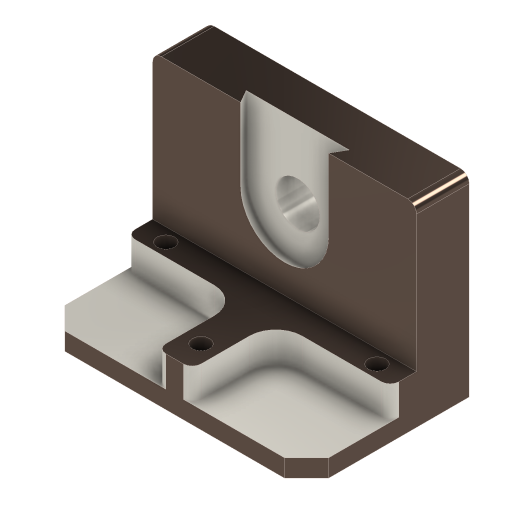
# Autodesk Inventor part: Part019. Corner block
Saved by Autodesk Inventor 2023.2 (Build 272271030, 271C)
## iProperties
Created: 2023-09-20
Part Number: Part019. Corner block
Material: Steel, Carbon
Document SubType Name: Modeling
Designer: User
Mass: 2416.08 g
Surface Area: 476.682 cm^2
Volume: 307.781 cm^3
Density: 7.85 g/cm^3
Appearance: Gunmetal - Antique Polished
Author: User
Autodesk Inventor part; units mm, degrees
ref_plane "YZ Plane" through (0, 0, 0) normal (1, 0, 0) x (0, 1, 0)
ref_plane "XZ Plane" through (0, 0, 0) normal (0, 1, 0) x (-1, 0, 0)
ref_plane "XY Plane" through (0, 0, 0) normal (0, 0, 1) x (1, 0, 0)
sketch "Sketch1" plane through (0, 0, 0) normal (0, 1, 0) x (-1, 0, 0)
  line L0 (60, -74) -> (-60, -74)
  line L1 (-60, -74) -> (-60, 0)
  line L2 (-60, 0) -> (60, 0)
  line L3 (60, 0) -> (60, -74)
  point P0 (0, 0)
  point P1 (0, 0)
  dimension "d0" = 120
  dimension "d1" = 74
  constraints: 8 end point, 2 parallel, 1 coincident, 1 horizontal, 1 midpoint, 1 perpendicular
  measures "d0" distance of L1.end L2.end
  measures "d1" distance of L0.end L1.end
extrude "Extrusion1" add sketch "Sketch1" along normal blind 8
chamfer "Chamfer1" distance 10 angle 45 2 edges at (60, 4, 0) (-60, 4, 0)
sketch "Sketch2" plane through (0, 8, 0) normal (0, 1, 0) x (1, 0, 0)
  line L0 (-50, 0) -> (-60, 10) projected
  line L1 (-50, 0) -> (50, 0) projected
  line L2 (60, 10) -> (60, 74) projected
  line L3 (60, 74) -> (-60, 74) projected
  line L4 (-60, 74) -> (-60, 10) projected
  line L5 (-60, 38) -> (-20, 38)
  line L6 (-8, 26) -> (-8, 0)
  line L7 (-8, 0) -> (-50, 0)
  line L8 (-60, 10) -> (-60, 38)
  arc A0 (-8, 26) -> (-20, 38) centre (-20, 26) ccw
  line L9 (0, 88.8) -> (0, -14.8) construction
  line L10 (50, 0) -> (60, 10)
  line L11 (60, 38) -> (20, 38)
  line L12 (8, 26) -> (8, 0)
  line L13 (8, 0) -> (50, 0)
  line L14 (60, 10) -> (60, 38)
  arc A1 (20, 38) -> (8, 26) centre (20, 26) ccw
  point P0 (0, 0)
  point P1 (8, 0)
  dimension "d7" = 12
  dimension "d8" = 38
  dimension "d9" = 16
  constraints: 18 end point, 9 symmetric about line, 6 point on line, 4 point on circle, 2 centre point, 2 parallel, 2 tangent, 1 horizontal, 1 perpendicular, 1 other
  measures "d7" radius of A0
  measures "d8" distance between parallel lines of L1 L5
  measures "d9" distance between parallel lines of L12 L6
extrude "Extrusion2" add sketch "Sketch2" along normal blind 14 contours L6 A0 L5 L4 L3 L2 L11 A1 L12 L1
sketch "Sketch3" plane through (0, 22, 0) normal (0, 1, 0) x (1, 0, 0)
  line L0 (-60, 74) -> (-60, 38) projected
  line L1 (60, 38) -> (60, 74) projected
  line L2 (60, 74) -> (-60, 74) projected
  line L3 (-60, 74) -> (-60, 10) projected
  line L4 (-60, 74) -> (60, 74)
  line L5 (60, 74) -> (60, 50)
  line L6 (60, 50) -> (-60, 50)
  line L7 (-60, 50) -> (-60, 74)
  point P0 (0, 0)
  point P1 (-60, 50)
  dimension "d12" = 24
  constraints: 8 end point, 2 parallel, 1 horizontal, 1 perpendicular, 1 point on line
  measures "d12" distance of L4.end L5.end
extrude "Extrusion3" add sketch "Sketch3" along normal blind 66
fillet "Fillet1" radius 4 6 edges at (60, 88, -62) (-60, 88, -62) (-60, 15, -38) (-8, 15, 0) (8, 15, 0) (60, 15, -38)
sketch "Sketch4" plane through (0, 88, 0) normal (0, 1, 0) x (1, 0, 0)
  line L0 (-56, 50) -> (56, 50) projected
  line L1 (-20, 50) -> (-23.4641, 56)
  line L2 (-23.4641, 56) -> (23.4641, 56)
  line L3 (60, 50) -> (-60, 50) projected
  line L4 (23.4641, 56) -> (20, 50)
  line L5 (0, 88.8) -> (0, -14.8) construction
  point P0 (0, 0)
  dimension "d16" = 60
  dimension "d17" = 40
  dimension "d18" = 6
  constraints: 6 end point, 2 point on line, 1 parallel, 1 other
  measures "d16" angle of L0 L1
  measures "d17" distance of L4.end L1.start
  measures "d18" distance between parallel lines of L0 L2
extrude "Extrusion4" cut sketch "Sketch4" against normal blind 33
sketch "Sketch5" plane through (0, 55, 0) normal (0, 1, 0) x (1, 0, 0)
  line L0 (-20, 50) -> (-23.4641, 56) projected
  line L1 (20, 50) -> (-20, 50) projected
  line L2 (-23.4641, 56) -> (23.4641, 56) projected
  line L3 (-20, 50) -> (0, 50)
  line L4 (60, 50) -> (-60, 50) projected
  line L5 (0, 50) -> (0, 56)
  line L6 (0, 56) -> (-23.4641, 56)
  point P0 (0, 0)
  constraints: 6 end point, 2 midpoint, 1 collinear
revolve "Revolution1" cut sketch "Sketch5" angle 360 about axis through (0, 55, -50) along (0, 0, -1)
sketch "Sketch6" plane through (-23.4641, 88, -56) normal (0, 0, 1) x (1, 0, 0)
  arc A0 (3.4641, -33) -> (43.4641, -33) centre (23.4641, -33) ccw projected
  point P0 (23.4641, -88)
  constraints: 1 coincident
hole "Hole1" at (0, 55, -56) direction (0, 0, -1) diameter 20 end through all
sketch "Sketch7" plane through (0, 22, 0) normal (0, 1, 0) x (1, 0, 0)
  line L0 (-4, 0) -> (4, 0) projected
  line L1 (-50, 0) -> (-4, 0) projected
  line L2 (0, 88.9657) -> (0, -15.7941) construction
  point P0 (0, 0)
  point P1 (-48, 44)
  point P2 (48, 44)
  point P3 (0, 12)
  point P4 (0, 0)
  dimension "d29" = 44
  dimension "d30" = 96
  dimension "d31" = 12
  constraints: 1 horizontal alignment, 1 midpoint, 1 symmetric about line, 1 vertical alignment
  measures "d29" distance from line of L1 point (-48, 44)
  measures "d30" distance of point (48, 44) point (-48, 44)
  measures "d31" distance from line of point (0, 12) L0
hole "Hole2" at (-48, 22, -44) at (48, 22, -44) at (0, 22, -12) direction (0, -1, 0) diameter 8 end through all
body "Solid1"
